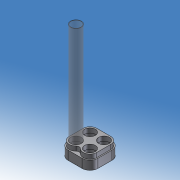
# Autodesk Inventor part: Flyspresso-CAD-files:_24W HOTEL
Saved by Autodesk Inventor 2015 SP1 (Build 190203100, 203)
## iProperties
RuleStatus: InUse
AfterDocSave0: file://Part Number Cleaner
Created: 2015-04-30
Material: Generic
Vendor: HHMI: JRC - ID&F
Document SubType Name: Modeling
Designer: JORDANJ
Density: 1 g/cm^3
Appearance: Default
DESIGN DEPARTMENT: HHMI: JRC - ID&F
ALTERED ITEM PART NUMBER: N/A
ALTERED ITEM VENDOR: N/A
ALTERED ITEM DESCRIPTION: N/A
Author: JORDANJ
Revision Number: 0
Autodesk Inventor part; units mm, degrees
ref_plane "YZ Plane" through (0, 0, 0) normal (1, 0, 0) x (0, 1, 0)
ref_plane "XY Plane" through (0, 0, 0) normal (0, 0, 1) x (1, 0, 0)
derived "_24W.ipt"
sketch "Well Profile" plane through (0, 0, 0) normal (0, 0, 1) x (1, 0, 0)
  line L0 (-7.2898, 57.65) -> (7.2898, 57.65) construction
  line L1 (7.2898, 57.65) -> (7.2898, 6.85) construction
  line L2 (7.2898, 6.85) -> (-7.2898, 6.85) construction
  line L3 (-7.2898, 6.85) -> (-7.2898, 57.65) construction
  line L4 (0, 57.65) -> (0, 6.85) construction
  line L5 (-6.731, 57.65) -> (-6.731, 6.85) construction
  line L6 (-8.6404, 17.5) -> (-8.3349, 0)
  line L7 (-8.3349, 0) -> (8.3349, 0)
  line L8 (8.3349, 0) -> (8.6404, 17.5)
  line L9 (-8.6404, 17.5) -> (8.6404, 17.5)
  line L10 (0, 17.5) -> (0, 0)
  line L11 (10.1404, 17.5) -> (27.4211, 17.5) construction
  line L12 (10.1404, 17.5) -> (10.4458, 0)
  line L13 (18.7807, 17.5) -> (18.7807, 0) construction
  line L14 (27.1156, 0) -> (27.4211, 17.5) construction
  line L15 (10.4458, 0) -> (27.1156, 0) construction
  line L16 (28.9211, 17.5) -> (46.2018, 17.5) construction
  line L17 (28.9211, 17.5) -> (29.2265, 0) construction
  line L18 (37.5614, 17.5) -> (37.5614, 0) construction
  line L19 (45.8963, 0) -> (46.2018, 17.5) construction
  line L20 (29.2265, 0) -> (45.8963, 0) construction
  line L21 (47.7018, 17.5) -> (64.9825, 17.5) construction
  line L22 (47.7018, 17.5) -> (48.0072, 0) construction
  line L23 (56.3421, 17.5) -> (56.3421, 0) construction
  line L24 (64.677, 0) -> (64.9825, 17.5) construction
  line L25 (48.0072, 0) -> (64.677, 0) construction
  line L26 (-14.6289, 17.5) -> (70.9711, 17.5)
  line L27 (70.9711, 17.5) -> (70.9711, -2.5)
  line L28 (70.9711, -2.5) -> (-14.6289, -2.5)
  line L29 (-14.6289, -2.5) -> (-14.6289, 17.5)
  line L30 (28.1711, 17.5) -> (28.1711, -2.5) construction
  line L31 (-14.6289, -2.5) -> (-14.2099, 9.5)
  line L32 (-10.1406, 17.5) -> (-9.8089, -1.5)
  line L33 (-9.8089, -1.5) -> (0, -1.5)
  line L34 (-14.6289, -2.5) -> (-13.128, -2.5)
  line L35 (0, -1.5) -> (0, 0)
  line L36 (-14.2099, 9.5) -> (-12.8583, 9.5)
  line L37 (-12.8583, 9.5) -> (-12.5789, 17.5)
  line L38 (-13.128, -2.5) -> (-12.7614, 8)
  line L39 (-11.4098, 8) -> (-12.7614, 8)
  line L40 (-11.1304, 16) -> (-10.1144, 16)
  line L41 (-11.078, 17.5) -> (-11.4098, 8)
  line L42 (-9.1404, 19.9885) -> (-8.7165, 19.9885)
  line L43 (-7.4982, 18.7913) -> (-7.179, 0.5)
  line L44 (-8.1436, 0.5) -> (-8.4626, 18.7744)
  line L45 (-8.7165, 19.024) -> (-9.1404, 19.024)
  line L46 (-9.1404, 19.024) -> (-9.1404, 19.9885)
  line L47 (-8.1436, 0.5) -> (-7.179, 0.5)
  line L48 (-8.3436, 0.5) -> (-6.0875, 0.5)
  line L49 (-6.0875, 0.5) -> (-6.0875, 0)
  line L50 (-7.0519, 0.5) -> (-7.4299, 22.1519)
  line L51 (-5.2526, 5.177) -> (-2.7637, 9.0605)
  line L52 (-1, 10.025) -> (-5.9549, 2.2938)
  line L53 (-6.0336, 2.0414) -> (-6.0875, 0.5)
  line L54 (-6.0875, 0.5) -> (-7.0519, 0.5)
  arc A0 (-5.9549, 2.2938) -> (-6.0336, 2.0414) centre (-5.5339, 2.024) ccw
  arc A1 (-6.1735, 5.4381) -> (-5.2526, 5.177) centre (-5.6736, 5.4468) ccw
  line L55 (-6.1735, 5.4381) -> (-6.4655, 22.1687)
  line L56 (-9.1404, 23.366) -> (-7.6838, 23.366)
  line L57 (8.1436, 0.5) -> (8.4626, 18.7744)
  line L58 (8.1436, 0.5) -> (7.179, 0.5)
  line L59 (7.4982, 18.7913) -> (7.179, 0.5)
  line L60 (7.0519, 0.5) -> (7.4299, 22.1519)
  line L61 (6.0875, 0.5) -> (7.0519, 0.5)
  line L62 (6.0336, 2.0414) -> (6.0875, 0.5)
  arc A2 (6.0336, 2.0414) -> (5.9549, 2.2938) centre (5.5339, 2.024) ccw
  line L63 (1, 10.025) -> (5.9549, 2.2938)
  arc A3 (5.2526, 5.177) -> (6.1735, 5.4381) centre (5.6736, 5.4468) ccw
  line L64 (5.2526, 5.177) -> (2.7637, 9.0605)
  line L65 (6.1735, 5.4381) -> (6.4655, 22.1687)
  line L66 (9.1404, 23.366) -> (7.6838, 23.366)
  line L67 (9.1404, 19.9885) -> (8.7165, 19.9885)
  line L68 (9.1404, 19.024) -> (9.1404, 19.9885)
  line L69 (8.7165, 19.024) -> (9.1404, 19.024)
  line L70 (9.3904, 17.5) -> (9.3904, -2.5) construction
  line L71 (-14.6289, 44.7236) -> (70.9711, 44.7236)
  line L72 (70.9711, 44.7236) -> (70.9711, 23.366)
  line L73 (70.9711, 23.366) -> (-14.6289, 23.366)
  line L74 (-14.6289, 23.366) -> (-14.6289, 44.7236)
  line L75 (-14.6289, 26.366) -> (70.9711, 26.366)
  line L76 (-5.9514, 36.526) -> (-4.3639, 36.526)
  line L77 (-4.3639, 36.526) -> (-4.3639, 7.2697)
  line L78 (-4.3639, 7.2697) -> (-5.9514, 7.2697)
  line L79 (-5.9514, 7.2697) -> (-5.9514, 36.526)
  line L80 (-5.1577, 36.526) -> (-5.1577, 7.2697)
  line L81 (-5.8244, 36.526) -> (-5.8244, 7.2697)
  line L82 (-51.6585, 0) -> (108.0006, 0) construction
  line L83 (0, -83.8923) -> (0, 101.204) construction
  line L84 (-14.6289, 37.526) -> (70.9711, 37.526)
  line L85 (-12.3429, 38.9484) -> (-9.6759, 38.9484)
  line L86 (-9.6759, 38.9484) -> (-9.6759, 37.526)
  line L87 (-9.6759, 37.526) -> (-12.3429, 37.526)
  line L88 (-12.3429, 37.526) -> (-12.3429, 38.9484)
  circle A4 centre (-11.0094, 38.0594) radius 0.889
  line L89 (-8.3327, 34.748) -> (-8.3327, 28.144)
  line L90 (-8.3327, 28.144) -> (-7.6977, 28.144)
  line L91 (-7.6977, 28.144) -> (-7.6977, 27.128)
  line L92 (-7.6977, 27.128) -> (-2.6177, 27.128)
  line L93 (-2.6177, 27.128) -> (-2.6177, 28.144)
  line L94 (-2.6177, 28.144) -> (-1.9827, 28.144)
  line L95 (-1.9827, 28.144) -> (-1.9827, 34.748)
  line L96 (-1.9827, 34.748) -> (-8.3327, 34.748)
  line L97 (-5.1577, 34.748) -> (-5.1577, 27.128)
  line L98 (-7.5707, 36.018) -> (-2.7447, 36.018)
  line L99 (-7.5707, 36.018) -> (-7.5707, 34.748)
  line L100 (-7.5707, 34.748) -> (-2.7447, 34.748)
  line L101 (-2.7447, 34.748) -> (-2.7447, 36.018)
  line L102 (-5.1577, 34.748) -> (-5.1577, 36.018)
  line L103 (8.3349, 0) -> (10.4458, 0)
  arc A5 (-1, 10.025) -> (-2.7637, 9.0605) centre (-1, 7.9302) ccw
  arc A6 (2.7637, 9.0605) -> (1, 10.025) centre (1, 7.9302) ccw
  line L104 (-1, 10.025) -> (1, 10.025)
  arc A7 (-8.4626, 18.7744) -> (-8.7165, 19.024) centre (-8.7165, 18.77) ccw
  arc A8 (-7.4982, 18.7913) -> (-8.7165, 19.9885) centre (-8.7165, 18.77) ccw
  arc A9 (8.7165, 19.024) -> (8.4626, 18.7744) centre (8.7165, 18.77) ccw
  arc A10 (8.7165, 19.9885) -> (7.4982, 18.7913) centre (8.7165, 18.77) ccw
  line L105 (-7.6838, 22.4015) -> (-9.1404, 22.4015)
  line L106 (-9.1404, 22.4015) -> (-9.1404, 23.366)
  line L107 (7.6838, 22.4015) -> (9.1404, 22.4015)
  line L108 (9.1404, 22.4015) -> (9.1404, 23.366)
  arc A11 (-7.4299, 22.1519) -> (-7.6838, 22.4015) centre (-7.6838, 22.1475) ccw
  arc A12 (7.6838, 22.4015) -> (7.4299, 22.1519) centre (7.6838, 22.1475) ccw
  arc A13 (-6.4655, 22.1687) -> (-7.6838, 23.366) centre (-7.6838, 22.1475) ccw
  arc A14 (7.6838, 23.366) -> (6.4655, 22.1687) centre (7.6838, 22.1475) ccw
  line L109 (8.6404, 17.5) -> (10.1404, 17.5)
  line L110 (-14.6289, 3.548) -> (70.9711, 3.548) construction
  line L111 (-14.6289, 15.976) -> (70.9711, 15.976) construction
  line L112 (-9.9202, 35.383) -> (-0.3952, 35.383)
  line L113 (-0.3952, 35.383) -> (-0.3952, 26.366) construction
  line L114 (-0.3952, 26.366) -> (-9.9202, 26.366)
  line L115 (-9.9202, 26.366) -> (-9.9202, 35.383) construction
  line L116 (-7.9517, 36.018) -> (-2.3637, 36.018)
  line L117 (-2.3637, 36.018) -> (-2.3637, 35.383)
  line L118 (-2.3637, 35.383) -> (-7.9517, 35.383)
  line L119 (-7.9517, 35.383) -> (-7.9517, 36.018)
  line L120 (-5.1577, 36.018) -> (-5.1577, 35.383)
  line L121 (-5.1577, 35.383) -> (-5.1577, 26.366)
  line L122 (-9.59, 35.383) -> (-9.59, 26.366)
  line L123 (-0.7254, 35.383) -> (-0.7254, 26.366)
  line L124 (-9.59, 28.9086) -> (-9.7678, 26.366)
  line L125 (-9.7678, 26.366) -> (-9.59, 26.366)
  line L126 (-9.59, 26.366) -> (-9.59, 28.9086)
  line L127 (-21.3289, -2.75) -> (77.6711, -2.75)
  line L128 (77.6711, -2.75) -> (77.6711, -57.45)
  line L129 (77.6711, -57.45) -> (-21.3289, -57.45)
  line L130 (-21.3289, -57.45) -> (-21.3289, -2.75)
  line L131 (-21.3289, 5.9) -> (77.6711, 5.9) construction
  line L132 (28.1711, -2.75) -> (28.1711, -57.45) construction
  line L133 (-5.9514, 36.526) -> (-4.3639, 36.526)
  line L134 (-4.3639, 36.526) -> (-4.0706, 36.018)
  line L135 (-4.0706, 36.018) -> (-6.2447, 36.018)
  line L136 (-6.2447, 36.018) -> (-5.9514, 36.526)
  line L137 (-5.1577, 36.526) -> (-5.1577, 36.018)
  line L138 (-5.9514, 37.526) -> (-5.8244, 37.526)
  line L139 (-5.8244, 37.526) -> (-5.8244, 36.526)
  line L140 (-5.8244, 36.526) -> (-5.9514, 36.526)
  line L141 (-5.9514, 36.526) -> (-5.9514, 37.526)
  line L142 (-12.5969, 38.8341) -> (-9.4219, 38.8341)
  line L143 (-9.4219, 38.8341) -> (-9.4219, 37.399)
  line L144 (-9.4219, 37.399) -> (-12.5969, 37.399)
  line L145 (-12.5969, 37.399) -> (-12.5969, 38.8341)
  line L146 (-12.4055, -1.5) -> (68.7476, -1.5)
  line L147 (68.7476, -1.5) -> (68.7476, -6.58)
  line L148 (68.7476, -6.58) -> (-12.4055, -6.58)
  line L149 (-12.4055, -6.58) -> (-12.4055, -1.5)
  point P0 (-7.5191, 19.9885)
  point P1 (-8.4669, 19.024)
  point P2 (-6.4864, 23.366)
  point P3 (8.4669, 19.024)
  point P4 (7.5191, 19.9885)
  point P5 (6.4864, 23.366)
  point P6 (-11.0094, 38.9484)
  point P7 (-11.0094, 38.8341)
  point P8 (28.1711, -1.5)
sketch "Microplate bottom" plane through (0, 0, 0) normal (0, 1, 0) x (-1, 0, 0)
  circle A0 centre (0, 0) radius 8.1403 construction
  line L0 (0, 14.6289) -> (-56.3421, 14.6289)
  line L1 (-70.9711, 0) -> (-70.9711, -109.7611)
  line L2 (-67.4711, -113.2611) -> (11.1289, -113.2611)
  line L3 (14.6289, -109.7611) -> (14.6289, 0)
  line L4 (13.7924, -46.9518) -> (-71.756, -46.9518) construction
  line L5 (-28.1711, -113.2611) -> (-28.1711, 14.6289) construction
  arc A1 (14.6289, 0) -> (0, 14.6289) centre (0, 0) ccw
  arc A2 (-56.3421, 14.6289) -> (-70.9711, 0) centre (-56.3421, 0) ccw
  arc A3 (-70.9711, -109.7611) -> (-67.4711, -113.2611) centre (-67.4711, -109.7611) ccw
  arc A4 (11.1289, -113.2611) -> (14.6289, -109.7611) centre (11.1289, -109.7611) ccw
  circle A5 centre (0, -18.7807) radius 8.1403 construction
  circle A6 centre (0, -37.5614) radius 8.1403 construction
  circle A7 centre (0, -56.3421) radius 8.1403 construction
  circle A8 centre (0, -75.1228) radius 8.1403 construction
  circle A9 centre (0, -93.9036) radius 8.1403 construction
  circle A10 centre (-18.7807, 0) radius 8.1403 construction
  circle A11 centre (-18.7807, -18.7807) radius 8.1403 construction
  circle A12 centre (-18.7807, -37.5614) radius 8.1403 construction
  circle A13 centre (-18.7807, -56.3421) radius 8.1403 construction
  circle A14 centre (-18.7807, -75.1228) radius 8.1403 construction
  circle A15 centre (-18.7807, -93.9036) radius 8.1403 construction
  circle A16 centre (-37.5614, 0) radius 8.1403 construction
  circle A17 centre (-37.5614, -18.7807) radius 8.1403 construction
  circle A18 centre (-37.5614, -37.5614) radius 8.1403 construction
  circle A19 centre (-37.5614, -56.3421) radius 8.1403 construction
  circle A20 centre (-37.5614, -75.1228) radius 8.1403 construction
  circle A21 centre (-37.5614, -93.9036) radius 8.1403 construction
  circle A22 centre (-56.3421, 0) radius 8.1403 construction
  circle A23 centre (-56.3421, -18.7807) radius 8.1403 construction
  circle A24 centre (-56.3421, -37.5614) radius 8.1403 construction
  circle A25 centre (-56.3421, -56.3421) radius 8.1403 construction
  circle A26 centre (-56.3421, -75.1228) radius 8.1403 construction
  circle A27 centre (-56.3421, -93.9036) radius 8.1403 construction
  circle A28 centre (-9.3904, -9.3904) radius 5.1397 construction
  line L6 (21.3289, -119.3161) -> (-77.6711, -119.3161)
  line L7 (-77.6711, -119.3161) -> (-77.6711, 22.6839)
  line L8 (-77.6711, 22.6839) -> (21.3289, 22.6839)
  line L9 (21.3289, 22.6839) -> (21.3289, -119.3161)
  line L10 (14.6289, -49.3161) -> (-70.9711, -49.3161) construction
  line L11 (21.3289, -48.3161) -> (-77.6711, -48.3161) construction
  line L12 (16.8289, -48.3161) -> (-73.1711, -48.3161) construction
  circle A29 centre (16.8289, -48.3161) radius 1.7
  circle A30 centre (-73.1711, -48.3161) radius 1.7
  arc A31 (21.3289, 19.6839) -> (18.3289, 22.6839) centre (18.3289, 19.6839) ccw
  point P0 (-70.9711, 0)
  point P1 (14.6289, 0)
  point P2 (-70.9711, -113.2611)
  point P3 (-70.9711, 14.6289)
  point P4 (14.6289, -113.2611)
  point P5 (-28.1711, -119.3161)
  point P6 (-28.1711, -48.3161)
sketch "Sketch63" plane through (0, 19.9885, 0) normal (0, 1, 0) x (1, 0, 0)
  circle A0 centre (0, 0) radius 8.7165
  circle A1 centre (0, 0) radius 9.1404 construction
  circle A2 centre (0, 18.7807) radius 8.7165
  circle A3 centre (0, 18.7807) radius 9.1404 construction
  circle A4 centre (18.7807, 0) radius 8.7165
  circle A5 centre (18.7807, 0) radius 9.1404 construction
  circle A6 centre (18.7807, 18.7807) radius 8.7165
  circle A7 centre (18.7807, 18.7807) radius 9.1404 construction
  line L0 (0, 27.9211) -> (18.7807, 27.9211)
  line L1 (27.9211, 18.7807) -> (27.9211, 0)
  line L2 (18.7807, -9.1404) -> (0, -9.1404)
  line L3 (-9.1404, 0) -> (-9.1404, 18.7807)
  arc A8 (0, 27.9211) -> (-9.1404, 18.7807) centre (0, 18.7807) ccw
  arc A9 (27.9211, 18.7807) -> (18.7807, 27.9211) centre (18.7807, 18.7807) ccw
  arc A10 (12.2309, -6.3754) -> (27.9211, 0) centre (18.7807, 0) ccw
  arc A11 (-9.1404, 0) -> (6.5498, -6.3754) centre (0, 0) ccw
  arc A12 (12.2309, -6.3754) -> (6.5498, -6.3754) centre (9.3904, -9.1404) ccw
  circle A13 centre (9.3904, 9.3904) radius 4.1396 construction
  circle A14 centre (9.3904, 9.3904) radius 3.714
sketch "Sketch2" plane through (0, 0, 0) normal (0, 0, 1) x (1, 0, 0)
  line L0 (-7.2898, 6.85) -> (-7.2898, 57.65) construction
  line L1 (-6.731, 57.65) -> (-6.731, 6.85) construction
  line L2 (7.2898, 57.65) -> (7.2898, 6.85) construction
  line L3 (0, 57.65) -> (0, 6.85) construction
  line L4 (-7.2898, 57.65) -> (7.2898, 57.65) construction
  line L5 (7.2898, 6.85) -> (-7.2898, 6.85) construction
  arc A0 (-7.4982, 18.7913) -> (-8.7165, 19.9885) centre (-8.7165, 18.77) ccw construction
  line L6 (-9.1404, 19.9885) -> (-8.7165, 19.9885) construction
  line L7 (-9.1404, 19.024) -> (-9.1404, 19.9885) construction
  line L8 (-8.7165, 19.024) -> (-9.1404, 19.024) construction
  arc A1 (-8.4626, 18.7744) -> (-8.7165, 19.024) centre (-8.7165, 18.77) ccw construction
  line L9 (-8.1436, 0.5) -> (-8.4626, 18.7744) construction
  arc A2 (8.7165, 19.9885) -> (7.4982, 18.7913) centre (8.7165, 18.77) ccw construction
  line L10 (9.1404, 19.9885) -> (8.7165, 19.9885) construction
  line L11 (9.1404, 19.024) -> (9.1404, 19.9885) construction
  line L12 (8.7165, 19.024) -> (9.1404, 19.024) construction
  arc A3 (8.7165, 19.024) -> (8.4626, 18.7744) centre (8.7165, 18.77) ccw construction
  line L13 (8.1436, 0.5) -> (8.4626, 18.7744) construction
  line L14 (7.4982, 18.7913) -> (7.179, 0.5) construction
  line L15 (8.1436, 0.5) -> (7.179, 0.5) construction
  line L16 (-8.1436, 0.5) -> (-7.179, 0.5) construction
  line L17 (18.7807, 17.5) -> (18.7807, 0) construction
  line L18 (0, 17.5) -> (0, 0) construction
  line L19 (-7.4982, 18.7913) -> (-7.179, 0.5) construction
  line L20 (-7.2898, 159.25) -> (7.2898, 159.25)
  line L21 (7.2898, 159.25) -> (7.2898, 6.85)
  line L22 (7.2898, 6.85) -> (-7.2898, 6.85)
  line L23 (-7.2898, 6.85) -> (-7.2898, 159.25)
  line L24 (0, 159.25) -> (0, 6.85)
  line L25 (-6.731, 6.85) -> (-6.731, 159.25)
  line L26 (-11.396, 24.65) -> (24.5976, 24.65)
  line L27 (24.5976, 24.65) -> (24.5976, 18.65)
  line L28 (24.5976, 18.65) -> (-11.396, 18.65)
  line L29 (-11.396, 18.65) -> (-11.396, 24.65)
  line L30 (8.3349, 0) -> (8.6404, 17.5) projected
  line L31 (10.1404, 17.5) -> (10.4458, 0) projected
  line L32 (8.3349, 0) -> (10.4458, 0) projected
  line L33 (8.6404, 17.5) -> (10.1404, 17.5) projected
  line L34 (8.418, 4.7625) -> (10.3627, 4.7625)
  line L35 (0, 0) -> (10.4458, 0)
  line L36 (10.4458, 0) -> (10.4458, -4.7625)
  line L37 (10.4458, -4.7625) -> (0, -4.7625)
  line L38 (0, -4.7625) -> (0, 0)
  point P0 (-7.2898, 83.05)
  dimension "d1" = 152.4
  dimension "d3" = 6
  dimension "d31" = 4.7625
  dimension "d32" = 9.525
  dimension "d33" = 4.7625
  dimension "d46" = 11.8
  constraints: 30 end point, 6 collinear, 6 parallel, 4 horizontal, 4 point on line, 3 midpoint, 3 perpendicular, 1 coincident, 1 vertical
  measures "d1" distance of L22.end L20.start
  measures "d3" distance of L28.end L26.start
  measures "d31" distance between parallel lines of L34 L32
  measures "d32" distance between parallel lines of L34 L37
  measures "d33" distance of L35.end L36.end
  measures "d46" distance between parallel lines of L22 L28
revolve "Revolution1" add sketch "Sketch2" angle 360 about axis through (0, 159.25, 0) along (0, -1, 0) contours L20 L25 L26 L23 | L26 L25 L28 L23 | L28 L25 L22 L23
ref_plane "Work Plane1" through (-11.396, 24.65, 0) normal (0, 1, 0) x (1, 0, 0)
sketch "Sketch4" plane through (-11.396, 24.65, 0) normal (0, 1, 0) x (1, 0, 0)
  circle A0 centre (11.396, 0) radius 7.2898 construction
  circle A1 centre (11.396, 0) radius 7.1628
  line L0 (11.396, 27.9171) -> (30.1767, 27.9171)
  line L1 (39.313, 18.7807) -> (39.313, 0)
  line L2 (30.1767, -9.1364) -> (11.396, -9.1364)
  line L3 (2.2596, 0) -> (2.2596, 18.7807)
  arc A2 (11.396, 27.9171) -> (2.2596, 18.7807) centre (11.396, 18.7807) ccw
  arc A3 (2.2596, 0) -> (17.9443, -6.3712) centre (11.396, 0) ccw
  arc A4 (23.6283, -6.3712) -> (39.313, 0) centre (30.1767, 0) ccw
  arc A5 (39.313, 18.7807) -> (30.1767, 27.9171) centre (30.1767, 18.7807) ccw
  circle A6 centre (11.396, 18.7807) radius 7.1628
  circle A7 centre (30.1767, 0) radius 7.1628
  circle A8 centre (30.1767, 18.7807) radius 7.1628
  line L4 (39.567, 113.2611) -> (39.567, -14.6289) construction
  arc A9 (23.6283, -6.3712) -> (17.9443, -6.3712) centre (20.7863, -9.1364) ccw
  dimension "d5" = 0.127
  dimension "d9" = 18.7807
  dimension "d12" = 18.7807
  dimension "d15" = 0.254
  constraints: 12 point on circle, 10 tangent, 9 centre point, 8 end point, 3 concentric, 3 equal radius, 2 horizontal, 2 parallel, 1 midpoint, 1 perpendicular, 1 vertical, 6 other
  measures "d5" radial gap between concentric circles of A0 A1
  measures "d9" distance of A0.centre A6.centre
  measures "d12" distance of A0.centre A7.centre
  measures "d15" distance between parallel lines of L4 L1
extrude "Extrusion1" add sketch "Sketch4" against normal blind 6 separate body contours L0 A5 L1 A4 A9 A3 L3 A2
revolve "Revolution2" add sketch "Sketch2" angle 360 about axis through (0, -4.7625, 0) along (0, 1, 0) contours L30 L34 L31 L32 | L32 L36 L37 L38 L35
pattern_linear "Rectangular Pattern1" count 2 spacing 18.7807 along (0, 0, -1) count 2 spacing 18.7807 along (1, 0, 0) of "Revolution2" bodies 3
sketch "Sketch7" plane through (18.7807, 4.7625, 0) normal (0, 1, 0) x (0.7071068, 0, 0.7071068)
  circle A0 centre (0, 0) radius 8.418 projected
  arc A1 (-9.7389, -3.5411) -> (-16.821, -3.5411) centre (-13.28, -13.28) ccw projected
  arc A2 (-16.821, -3.5411) -> (-16.821, 3.5411) centre (-26.5599, 0) ccw projected
  arc A3 (-16.821, 3.5411) -> (-9.7389, 3.5411) centre (-13.28, 13.28) ccw projected
  arc A4 (-9.7389, 3.5411) -> (-9.7389, -3.5411) centre (0, 0) ccw projected
  circle A5 centre (-26.5599, 0) radius 8.418 projected
  circle A6 centre (-13.28, 13.28) radius 8.418 projected
  circle A7 centre (-13.28, -13.28) radius 8.418 projected
  arc A8 (-3.5411, -9.7389) -> (-3.5411, 9.7389) centre (0, 0) ccw projected
  arc A9 (-3.5411, 9.7389) -> (-23.0189, 9.7389) centre (-13.28, 13.28) ccw projected
  arc A10 (-23.0189, 9.7389) -> (-23.0189, -9.7389) centre (-26.5599, 0) ccw projected
  arc A11 (-23.0189, -9.7389) -> (-3.5411, -9.7389) centre (-13.28, -13.28) ccw projected
  line L0 (-33.9462, 7.3863) -> (-20.6663, 20.6663)
  line L1 (-5.8937, 20.6663) -> (7.3863, 7.3863)
  line L2 (7.3863, -7.3863) -> (-5.8937, -20.6663)
  line L3 (-20.6663, -20.6663) -> (-33.9462, -7.3863)
  arc A12 (-5.8937, 20.6663) -> (-20.6663, 20.6663) centre (-13.28, 13.28) ccw
  arc A13 (7.3863, -7.3863) -> (7.3863, 7.3863) centre (0, 0) ccw
  arc A14 (-20.6663, -20.6663) -> (-5.8937, -20.6663) centre (-13.28, -13.28) ccw
  arc A15 (-33.9462, 7.3863) -> (-33.9462, -7.3863) centre (-26.5599, 0) ccw
  arc A16 (-3.4045, 9.8754) -> (-23.1554, 9.8754) centre (-13.28, 13.28) ccw projected
  arc A17 (-3.4045, -9.8754) -> (-3.4045, 9.8754) centre (0, 0) ccw projected
  arc A18 (-23.1554, -9.8754) -> (-3.4045, -9.8754) centre (-13.28, -13.28) ccw projected
  constraints: 8 end point, 8 point on circle, 8 tangent, 4 centre point, 4 equal radius, 3 concentric, 2 parallel, 1 perpendicular
extrude "Extrusion4" add sketch "Sketch7" against normal up to surface (9.525 mm away) contours A1 A2 A3 A4 | L0 A12 A16 A17 A13 A18 A14 L3 A15 | L1 A17 A16 | A18 A17 L2 bodies 3
extrude "Extrusion5" cut sketch "Sketch63" against normal through all contours A0 | A2 | A4 | A6 | L0 A9 L1 A10 A12 A11 L3 A8 | A11 A12 A10 L2 | A14 keep common part bodies 3
sketch "Sketch8" plane through (-11.396, 18.65, 0) normal (0, -1, 0) x (1, 0, 0)
  circle A0 centre (30.1767, -18.7807) radius 7.1628 construction
  circle A1 centre (30.1767, 0) radius 7.1628 construction
  circle A2 centre (11.396, -18.7807) radius 7.1628 construction
  circle A3 centre (11.396, 0) radius 7.1628 construction
  arc A4 (2.2596, -18.7807) -> (11.396, -27.9171) centre (11.396, -18.7807) ccw construction
  line L0 (11.396, -27.9171) -> (30.1767, -27.9171) construction
  arc A5 (30.1767, -27.9171) -> (39.313, -18.7807) centre (30.1767, -18.7807) ccw construction
  line L1 (39.313, -18.7807) -> (39.313, 0) construction
  arc A6 (39.313, 0) -> (23.6283, 6.3712) centre (30.1767, 0) ccw construction
  arc A7 (17.9443, 6.3712) -> (23.6283, 6.3712) centre (20.7863, 9.1364) ccw construction
  arc A8 (17.9443, 6.3712) -> (2.2596, 0) centre (11.396, 0) ccw construction
  line L2 (2.2596, 0) -> (2.2596, -18.7807) construction
  circle A9 centre (11.396, 0) radius 7.4168
  circle A10 centre (30.1767, 0) radius 7.4168
  circle A11 centre (30.1767, -18.7807) radius 7.4168
  circle A12 centre (11.396, -18.7807) radius 7.4168
  line L3 (11.396, 10.5918) -> (30.1767, 10.5918)
  line L4 (40.7685, 0) -> (40.7685, -18.7807)
  line L5 (30.1767, -29.3725) -> (11.396, -29.3725)
  line L6 (0.8042, -18.7807) -> (0.8042, 0)
  arc A13 (11.396, 10.5918) -> (0.8042, 0) centre (11.396, 0) ccw
  arc A14 (40.7685, 0) -> (30.1767, 10.5918) centre (30.1767, 0) ccw
  arc A15 (30.1767, -29.3725) -> (40.7685, -18.7807) centre (30.1767, -18.7807) ccw
  arc A16 (0.8042, -18.7807) -> (11.396, -29.3725) centre (11.396, -18.7807) ccw
  dimension "d47" = 0.254
  dimension "d49" = 3.175
  constraints: 8 centre point, 8 end point, 8 point on circle, 8 tangent, 6 equal radius, 2 concentric, 2 parallel, 1 horizontal, 1 perpendicular
  measures "d47" radial gap between concentric circles of A3 A9
  measures "d49" radial gap between concentric circles of A9 A13
extrude "Extrusion6" add sketch "Sketch8" along normal up to surface (11.8 mm away) from surface at 0 separate body
equation "\"d31\" = d33"
equation "\"d9\" = microplate_well_spacing"
equation "\"d12\" = microplate_well_spacing"
equation "\"d16\" = d3"
equation "\"d37\" = microplate_well_spacing"
equation "\"d40\" = microplate_well_spacing"
equation "\"microplate_well_spacing\" = 18.78071"
